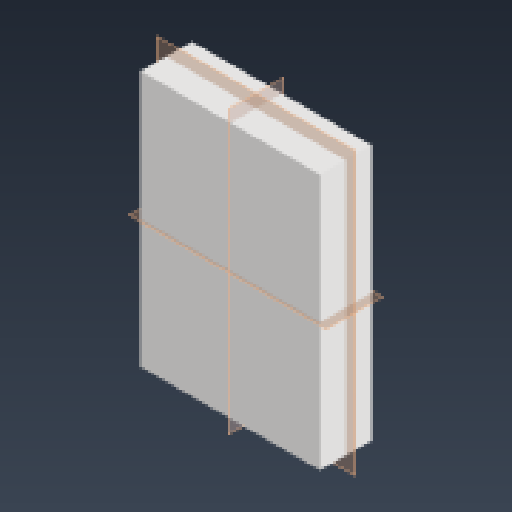
# Autodesk Inventor part: Козырёк_версия_2
Saved by Autodesk Inventor 2023.2 (Build 272271030, 271C)
## iProperties
Created: 2025-10-07
Part Number: Козырёк_версия_2
Material: Типовые
Document SubType Name: Modeling
Designer: Олег Коноваленко
Density: 1 g/cm^3
Appearance: По умолчанию
Author: Олег Коноваленко
Autodesk Inventor part; units mm, degrees
sketch "Эскиз1" plane through (0, 0, 0) normal (0, 0, 1) x (1, 0, 0)
  arc A0 (-20, -20) -> (-10, -30) centre (-10, -20) ccw projected
  line L0 (-20, 20) -> (-20, -20) projected
  arc A1 (-10, 30) -> (-20, 20) centre (-10, 20) ccw projected
  line L1 (10, 30) -> (-10, 30) projected
  arc A2 (20, 20) -> (10, 30) centre (10, 20) ccw projected
  line L2 (20, -20) -> (20, 20) projected
  arc A3 (10, -30) -> (20, -20) centre (10, -20) ccw projected
  line L3 (-10, -30) -> (10, -30) projected
  arc A4 (10, -35) -> (25, -20) centre (10, -20) ccw
  line L4 (25, -20) -> (25, 20)
  arc A5 (25, 20) -> (10, 35) centre (10, 20) ccw
  line L5 (10, 35) -> (-10, 35)
  arc A6 (-10, 35) -> (-25, 20) centre (-10, 20) ccw
  line L6 (-25, 20) -> (-25, -20)
  arc A7 (-25, -20) -> (-10, -35) centre (-10, -20) ccw
  line L7 (-10, -35) -> (10, -35)
  dimension "d4" = 5
  constraints: 8 end point, 8 point on circle, 4 centre point, 7 other
  measures "d4" distance between parallel lines of L3 L7
extrude "Выдавливание1" add sketch "Эскиз1" along normal mid plane 30
